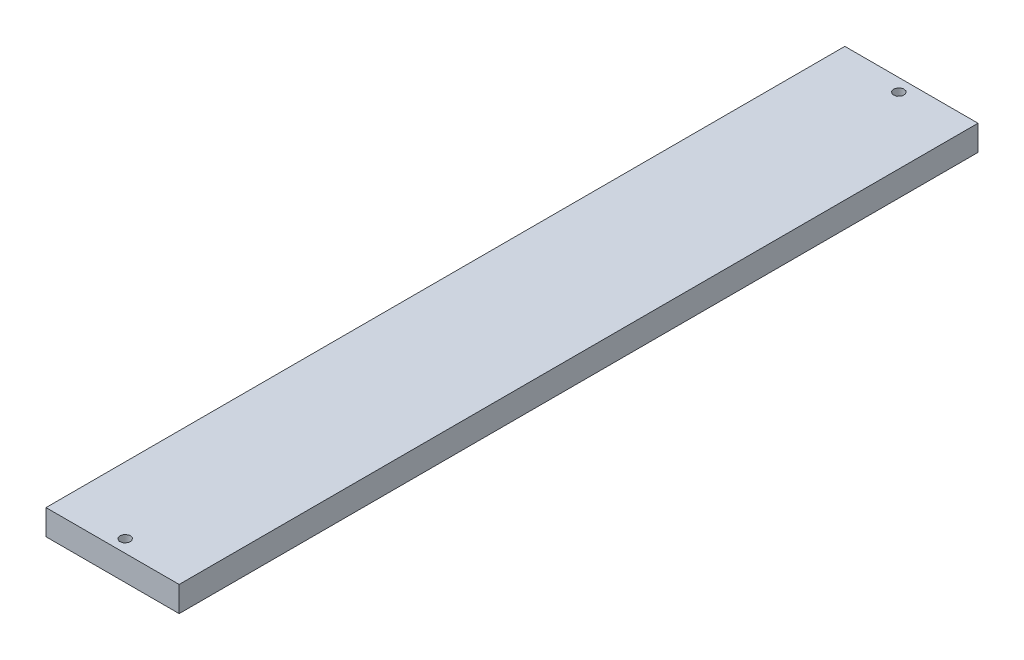
# Autodesk Inventor part: J
Saved by Autodesk Inventor 2024 (Build 280153000, 153)
## iProperties
Created: 2024-03-20
Part Number: J
Material: Generic
Document SubType Name: Modeling
Designer: marco
Density: 1 g/cm^3
Appearance: Wood - Painted White
Author: marco
Autodesk Inventor part; units mm, degrees
ref_plane "YZ Plane" through (0, 0, 0) normal (1, 0, 0) x (0, 1, 0)
ref_plane "XZ Plane" through (0, 0, 0) normal (0, 1, 0) x (-1, 0, 0)
ref_plane "XY Plane" through (0, 0, 0) normal (0, 0, 1) x (1, 0, 0)
sketch "Sketch1" plane through (0, 0, 0) normal (0, 1, 0) x (-1, 0, 0)
  line L0 (50, 300) -> (-50, 300)
  line L1 (-50, 300) -> (-50, -300)
  line L2 (-50, -300) -> (50, -300)
  line L3 (50, -300) -> (50, 300)
  line L4 (0, 300) -> (0, 290.5)
  line L5 (0, -300) -> (0, -290.5)
  circle A0 centre (0, -290.5) radius 4
  circle A1 centre (0, 290.5) radius 4
  dimension "d0" = 100
  dimension "d1" = 600
  dimension "d2" = 9.5
  dimension "d3" = 9.5
  dimension "d4" = 8
  dimension "d5" = 8
  constraints: 12 end point, 2 centre point, 2 coincident, 2 midpoint, 2 parallel, 2 vertical, 1 horizontal, 1 perpendicular
  measures "d0" distance of L2.end L1.end
  measures "d1" distance of L1.end L0.end
  measures "d2" distance of L4.start L4.end
  measures "d3" distance of L5.start L5.end
  measures "d4" diameter of A0
  measures "d5" diameter of A1
extrude "Extrusion1" add sketch "Sketch1" along normal mid plane 19
body "Solid1"
